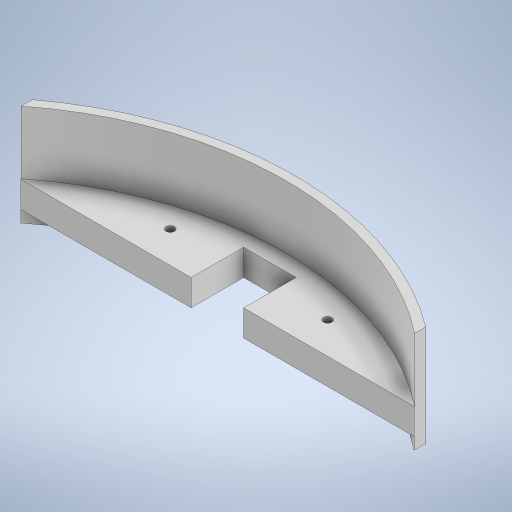
# Autodesk Inventor part: 中間台2
Saved by Autodesk Inventor 2023 (Build 270158000, 158)
## iProperties
Created: 2022-12-03
Part Number: 中間台2
Material: 一般
Document SubType Name: Modeling
Designer: RiSA
Density: 1 g/cm^3
Appearance: 既定
Author: RiSA
Autodesk Inventor part; units mm, degrees
ref_plane "YZ Plane" through (0, 0, 0) normal (1, 0, 0) x (0, 1, 0)
ref_plane "XZ Plane" through (0, 0, 0) normal (0, 1, 0) x (-1, 0, 0)
ref_plane "XY Plane" through (0, 0, 0) normal (0, 0, 1) x (1, 0, 0)
sketch "スケッチ1" plane through (0, 0, 0) normal (0, 1, 0) x (-1, 0, 0)
  circle A0 centre (0, 0) radius 125
  dimension "d0" = 250
  constraints: 1 centre point, 1 coincident
  measures "d0" diameter of A0
extrude "押し出し1" add sketch "スケッチ1" along normal blind 4
sketch "スケッチ2" plane through (0, 4, 0) normal (0, 1, 0) x (1, 0, 0)
  line L0 (75, -84.411) -> (-75, -84.411)
  line L1 (-75, -84.411) -> (-75, 95.589)
  line L2 (-75, 95.589) -> (75, 95.589)
  line L3 (75, 95.589) -> (75, -84.411)
  line L4 (75, -84.411) -> (-75, 95.589) construction
  line L5 (-75, -84.411) -> (75, 95.589) construction
  circle A0 centre (0, 0) radius 121.5
  line L6 (0, 0) -> (0, -125) construction
  circle A1 centre (0, 0) radius 125 projected
  line L7 (0, 0) -> (108.2532, 62.5) construction
  line L8 (0, 0) -> (-108.2532, 62.5) construction
  line L9 (-75, 95.589) -> (-75, 100)
  line L10 (75, 95.589) -> (75, 100)
  point P0 (0, 5.589)
  dimension "d3" = 150
  dimension "d4" = 180
  dimension "d5" = 243
  dimension "d8" = 360
  constraints: 22 end point, 5 point on circle, 3 parallel, 2 midpoint, 2 perpendicular, 1 centre point, 1 coincident, 1 horizontal, 1 vertical, 10 other
  measures "d3" distance of L1.end L2.end
  measures "d4" distance of L0.end L1.end
  measures "d5" diameter of A0
extrude "押し出し2" cut sketch "スケッチ2" against normal blind 10 contours L3 A0 L1 L0 | L10 A1 L9 A0 picked at (-95.605, -76.597)
sketch "スケッチ4" plane through (0, 0, 0) normal (0, -1, 0) x (1, 0, 0)
  circle A0 centre (0, 0) radius 121.5
  line L0 (75, 84.411) -> (75, -100) projected
  line L1 (75, -95.589) -> (-75, -95.589)
  line L2 (-75, -100) -> (-75, 84.411) projected
  dimension "d13" = 243
  constraints: 2 end point, 2 point on circle, 2 point on line, 1 centre point, 1 coincident
  measures "d13" diameter of A0
sketch "スケッチ5" plane through (0, 0, 0) normal (0, -1, 0) x (1, 0, 0)
  circle A0 centre (0, 0) radius 121.5
  line L0 (75, -100) -> (75, 84.411) projected
  line L1 (72, -97.8685) -> (72, -67.8685)
  line L2 (72, -67.8685) -> (42, -67.8685)
  line L3 (42, -67.8685) -> (42, -114.0099)
  line L4 (0, -79.2159) -> (0, -106.232)
  line L5 (-72, -97.8685) -> (-72, -67.8685)
  line L6 (-72, -67.8685) -> (-42, -67.8685)
  line L7 (-42, -67.8685) -> (-42, -114.0099)
  point P0 (72, -91.7633)
  point P1 (-72, -91.7633)
  point P2 (-75, -100)
  dimension "d14" = 243
  dimension "d15" = 3
  dimension "d16" = 30
  dimension "d17" = 30
  constraints: 14 end point, 6 symmetric about line, 2 perpendicular, 2 point on circle, 2 vertical, 1 centre point, 1 coincident
  measures "d14" diameter of A0
  measures "d15" distance from line of L0 point (72, -91.763)
  measures "d16" distance of L1.start L1.end
  measures "d17" distance of L1.end L2.end
extrude "押し出し3" add sketch "スケッチ5" along normal blind 10 contours L5 L6 L7 A0 | A0 L3 L2 L1
sketch "スケッチ6" plane through (0, 0, 0) normal (0, -1, 0) x (1, 0, 0)
  circle A0 centre (0, 0) radius 125
  circle A1 centre (0, 0) radius 121.5
  arc A2 (-75, -100) -> (75, -100) centre (0, 0) ccw projected
  line L0 (75, -100) -> (75, -95.589)
  line L1 (75, -100) -> (75, 84.411) projected
  line L2 (-75, -100) -> (-75, -95.589)
  line L3 (-75, 84.411) -> (-75, -100) projected
  dimension "d20" = 243
  constraints: 4 end point, 3 point on circle, 2 centre point, 2 coincident, 2 point on line
  measures "d20" diameter of A1
extrude "押し出し4" add sketch "スケッチ6" along normal blind 15 contours L2 A1 L0 A0 picked at (70.9725, -99.8432)
sketch "スケッチ7" plane through (0, 4, 0) normal (0, 1, 0) x (1, 0, 0)
  circle A0 centre (0, 0) radius 125
  circle A1 centre (0, 0) radius 121.5
  arc A2 (-72, 97.8685) -> (-75, 95.589) centre (0, 0) ccw projected
  line L0 (-75, 95.589) -> (-75, 100)
  line L1 (-75, 100) -> (-75, -84.411) projected
  line L2 (-75, 95.589) -> (-75, 100)
  line L3 (75, -84.411) -> (75, 100) projected
  line L4 (75, 95.589) -> (75, 100)
  dimension "d23" = 250
  dimension "d24" = 243
  constraints: 6 end point, 2 centre point, 2 coincident, 1 collinear, 1 point on circle, 1 point on line
  measures "d23" diameter of A0
  measures "d24" diameter of A1
extrude "押し出し5" add sketch "スケッチ7" along normal blind 15 contours L3 A1 L0 A0 picked at (71.0701, 99.7839)
sketch "スケッチ8" plane through (0, -10, 0) normal (0, -1, 0) x (1, 0, 0)
  line L0 (75, -100) -> (75, -95.589) projected
  line L1 (42, -67.8685) -> (75, -67.8685)
  line L2 (75, -67.8685) -> (75, -95.589)
  line L3 (75, -95.589) -> (42, -95.589)
  line L4 (42, -95.589) -> (42, -67.8685)
  line L5 (0, 0) -> (0, -35.3892)
  line L6 (-75, -100) -> (-75, -95.589)
  line L7 (-42, -67.8685) -> (-75, -67.8685)
  line L8 (-75, -67.8685) -> (-75, -95.589)
  line L9 (-75, -95.589) -> (-42, -95.589)
  line L10 (-42, -95.589) -> (-42, -67.8685)
  constraints: 20 end point, 5 symmetric about line, 2 parallel, 1 horizontal, 1 perpendicular, 1 vertical
extrude "押し出し6" cut sketch "スケッチ8" against normal blind 10
sketch "スケッチ9" plane through (0, -10, 0) normal (0, -1, 0) x (1, 0, 0)
  line L0 (72, -95.589) -> (42, -95.589) projected
  line L1 (42, -95.589) -> (72, -95.589)
  line L2 (72, -95.589) -> (72, -97.589)
  line L3 (72, -97.589) -> (42, -97.589)
  line L4 (42, -97.589) -> (42, -95.589)
  line L5 (0, 0) -> (0, -14.9352)
  line L6 (-72, -95.589) -> (-42, -95.589)
  line L7 (-42, -95.589) -> (-72, -95.589)
  line L8 (-72, -95.589) -> (-72, -97.589)
  line L9 (-72, -97.589) -> (-42, -97.589)
  line L10 (-42, -97.589) -> (-42, -95.589)
  dimension "d29" = 30
  dimension "d30" = 2
  constraints: 20 end point, 5 symmetric about line, 2 parallel, 1 horizontal, 1 perpendicular, 1 vertical
  measures "d29" distance of L2.end L3.end
  measures "d30" distance of L1.end L2.end
extrude "押し出し7" cut sketch "スケッチ9" against normal blind 10
extrude "押し出し8" add sketch "スケッチ4" along normal blind 10 contours L1 A0 picked at (-20.9725, -98.3728)
sketch "スケッチ12" plane through (0, 4, 0) normal (0, 1, 0) x (1, 0, 0)
  circle A0 centre (0, 0) radius 121.5
  dimension "d35" = 243
  constraints: 1 centre point, 1 coincident
  measures "d35" diameter of A0
extrude "押し出し9" cut sketch "スケッチ12" against normal blind 4
sketch "スケッチ13" plane through (0, -10, 0) normal (0, -1, 0) x (1, 0, 0)
  line L0 (75, -95.589) -> (-75, -95.589) projected
  line L1 (0, -112.5559) -> (0, -100.6989)
  point P0 (0, 0)
  point P1 (0, -107.589)
  point P2 (-30, -107.589)
  point P3 (30, -107.589)
  dimension "d38" = 12
  dimension "d39" = 30
  constraints: 2 end point, 1 symmetric about line, 1 vertical
  measures "d38" distance from line of point (0, -107.589) L0
  measures "d39" distance of point (0, -107.589) point (-30, -107.589)
hole "穴1" at (-30, -10, -107.589) at (0, -10, -107.589) at (30, -10, -107.589) direction (0, 1, 0) diameter 3.2 end through all
sketch "スケッチ14" plane through (0, 19, 0) normal (0, 1, 0) x (1, 0, 0)
  circle A0 centre (0, 0) radius 121.5
  circle A1 centre (0, 0) radius 121.65
  line L0 (-75, 95.589) -> (75, 95.589) projected
  line L1 (-75, 95.589) -> (-75, 95.7796)
  line L2 (-75, 95.589) -> (-75, 100) projected
  arc A2 (75, 95.589) -> (-75, 95.589) centre (0, 0) ccw projected
  line L3 (75, 95.589) -> (75, 95.7796)
  line L4 (75, 95.589) -> (75, 100) projected
  dimension "d47" = 243
  dimension "d48" = 243.3
  constraints: 4 end point, 2 centre point, 2 coincident, 2 point on circle, 2 point on line
  measures "d47" diameter of A0
  measures "d48" diameter of A1
extrude "押し出し10" cut sketch "スケッチ14" against normal blind 19
sketch "スケッチ15" plane through (0, 19, 0) normal (0, 1, 0) x (1, 0, 0)
  circle A0 centre (0, 0) radius 121.65
  circle A1 centre (0, 0) radius 125
  line L0 (-75, 95.589) -> (-75, 100) projected
  line L1 (-75, 100) -> (-75, 95.589)
  arc A2 (75, 100) -> (-75, 100) centre (0, 0) ccw projected
  line L2 (-75, 95.589) -> (75, 95.589) projected
  line L3 (75, 100) -> (75, 95.589)
  point P0 (-75, 95.7796)
  point P1 (75, 95.7796)
  dimension "d51" = 243.3
  dimension "d52" = 250
  constraints: 4 end point, 2 coincident, 1 centre point, 1 collinear, 1 perpendicular, 2 other
  measures "d52" diameter of A1
extrude "押し出し11" add sketch "スケッチ15" along normal blind 5 contours A0 L0 A1 L3 picked at (-70.971, 99.9661)
sketch "スケッチ16" plane through (0, 0, 0) normal (0, 1, 0) x (1, 0, 0)
  line L0 (10, 75.589) -> (-10, 75.589)
  line L1 (-10, 75.589) -> (-10, 115.589)
  line L2 (-10, 115.589) -> (10, 115.589)
  line L3 (10, 115.589) -> (10, 75.589)
  line L4 (75, 95.589) -> (-75, 95.589) projected
  line L5 (10, 75.589) -> (-10, 115.589) construction
  line L6 (-10, 75.589) -> (10, 115.589) construction
  point P0 (0, 0)
  point P1 (0, 95.589)
  dimension "d55" = 20
  dimension "d56" = 40
  constraints: 12 end point, 3 midpoint, 2 parallel, 1 horizontal, 1 perpendicular
  measures "d55" distance of L1.end L2.end
  measures "d56" distance of L0.end L1.end
extrude "押し出し12" cut sketch "スケッチ16" against normal blind 20
sketch "スケッチ17" plane through (0, -15, 0) normal (0, -1, 0) x (1, 0, 0)
  line L0 (-10, -95.589) -> (-75, -95.589) projected
  line L1 (-75, -95.589) -> (75, -95.589)
  line L2 (75, -95.589) -> (75, -127.9303)
  line L3 (75, -127.9303) -> (-75, -127.9303)
  line L4 (-75, -127.9303) -> (-75, -95.589)
  point P0 (0, 0)
  constraints: 8 end point, 2 parallel, 1 horizontal, 1 perpendicular
extrude "押し出し13" cut sketch "スケッチ17" against normal blind 0.5
